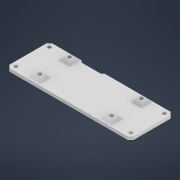
# Autodesk Inventor part: VFD_Mount
Saved by Autodesk Inventor 2021.1 (Build 251245010, 245A)
## iProperties
Created: 2020-11-26
Part Number: VFD_Mount
Material: Generic
Document SubType Name: Modeling
Designer: Alex
Density: 1 g/cm^3
Appearance: Default
Author: Alex
Autodesk Inventor part; units mm, degrees
ref_plane "YZ Plane" through (0, 0, 0) normal (1, 0, 0) x (0, 1, 0)
ref_plane "XZ Plane" through (0, 0, 0) normal (0, 1, 0) x (-1, 0, 0)
ref_plane "XY Plane" through (0, 0, 0) normal (0, 0, 1) x (1, 0, 0)
sketch "Sketch1" plane through (0, 0, 0) normal (0, 1, 0) x (-1, 0, 0)
  line L0 (64.8, -22.3) -> (-64.8, -22.3)
  line L1 (-64.8, -22.3) -> (-64.8, 22.3)
  line L2 (-64.8, 22.3) -> (64.8, 22.3)
  line L3 (64.8, 22.3) -> (64.8, -22.3)
  point P0 (0, 0)
  point P1 (64.8, 0)
  point P2 (0, -22.3)
  dimension "d0" = 129.6
  dimension "d1" = 44.6
  constraints: 8 end point, 2 midpoint, 2 parallel, 1 horizontal, 1 horizontal alignment, 1 perpendicular, 1 vertical alignment
  measures "d0" distance of L0.start L0.end
  measures "d1" distance of L2.end L0.start
extrude "Extrusion1" add sketch "Sketch1" along normal blind 3
sketch "Sketch2" plane through (0, 3, 0) normal (0, 1, 0) x (1, 0, 0)
  line L0 (-64.8, -22.3) -> (64.8, -22.3) construction
  line L1 (64.8, -22.3) -> (64.8, 22.3) construction
  line L2 (64.8, 22.3) -> (-64.8, 22.3) construction
  line L3 (-64.8, 22.3) -> (-64.8, -22.3) construction
  line L4 (-40, 18.55) -> (40, 18.55) construction
  line L5 (40, 18.55) -> (40, -17.45) construction
  line L6 (40, -17.45) -> (-40, -17.45) construction
  line L7 (-40, -17.45) -> (-40, 18.55) construction
  circle A0 centre (-37.5, 16.05) radius 1.25 construction
  circle A1 centre (37.5, 16.05) radius 1.25 construction
  circle A2 centre (37.5, -14.95) radius 1.25 construction
  circle A3 centre (-37.5, -14.95) radius 1.25 construction
  line L8 (-37.5, 12.5) -> (37.5, 12.5) construction
  line L9 (37.5, 12.5) -> (37.5, -12.5) construction
  line L10 (37.5, -12.5) -> (-37.5, -12.5) construction
  line L11 (-37.5, -12.5) -> (-37.5, 12.5) construction
  line L12 (-40, 18.55) -> (-35, 18.55)
  line L13 (-35, 18.55) -> (-35, 13.55)
  line L14 (-35, 13.55) -> (-40, 13.55)
  line L15 (-40, 13.55) -> (-40, 18.55)
  line L16 (-40, 18.55) -> (-35, 13.55) construction
  line L17 (-35, 18.55) -> (-40, 13.55) construction
  line L18 (35, 18.55) -> (40, 18.55)
  line L19 (40, 18.55) -> (40, 13.55)
  line L20 (40, 13.55) -> (35, 13.55)
  line L21 (35, 13.55) -> (35, 18.55)
  line L22 (35, 18.55) -> (40, 13.55) construction
  line L23 (40, 18.55) -> (35, 13.55) construction
  line L24 (35, -12.45) -> (40, -12.45)
  line L25 (40, -12.45) -> (40, -17.45)
  line L26 (40, -17.45) -> (35, -17.45)
  line L27 (35, -17.45) -> (35, -12.45)
  line L28 (35, -12.45) -> (40, -17.45) construction
  line L29 (40, -12.45) -> (35, -17.45) construction
  line L30 (-40, -12.45) -> (-35, -12.45)
  line L31 (-35, -12.45) -> (-35, -17.45)
  line L32 (-35, -17.45) -> (-40, -17.45)
  line L33 (-40, -17.45) -> (-40, -12.45)
  line L34 (-40, -12.45) -> (-35, -17.45) construction
  line L35 (-35, -12.45) -> (-40, -17.45) construction
  point P0 (0, 0)
  point P1 (0, 12.5)
  point P2 (0, 22.3)
  dimension "d4" = 80
  dimension "d5" = 36
  dimension "d6" = 2.5
  dimension "d7" = 2.5
  dimension "d8" = 2.5
  dimension "d9" = 2.5
  dimension "d10" = 2.5
  dimension "d12" = 75
  dimension "d13" = 25
  dimension "d14" = 2.5
  dimension "d15" = 4.95
  dimension "d16" = 9.8
  dimension "d17" = 5
  constraints: 64 end point, 12 parallel, 10 midpoint, 7 equal length, 6 horizontal, 6 perpendicular, 4 centre point, 3 equal radius, 3 vertical alignment, 2 horizontal alignment
  measures "d4" distance of L5.end L6.end
  measures "d5" distance of L4.end L5.end
  measures "d6" diameter of A0
  measures "d7" distance from line of L7 A0.centre
  measures "d8" distance from line of A1.centre L5
  measures "d9" distance from line of L4 A0.centre
  measures "d10" distance from line of L6 A3.centre
  measures "d12" distance of L8.start L8.end
  measures "d13" distance of L10.end L8.start
  measures "d14" distance between parallel lines of L7 L11
  measures "d15" distance between parallel lines of L10 L6
  measures "d16" distance between parallel lines of L10 L0
  measures "d17" distance of L12.end L13.end
extrude "Extrusion2" add sketch "Sketch2" along normal blind 3
sketch "Sketch3" plane through (0, 6, 0) normal (0, 1, 0) x (1, 0, 0)
  line L0 (-35, 18.55) -> (-40, 13.55) construction
  point P0 (0, 0)
  point P1 (-37.5, -14.95)
  point P2 (-37.5, 16.05)
  point P3 (37.5, 16.05)
  point P4 (37.5, -14.95)
hole "Hole1" at (-37.5, 6, 14.95) at (-37.5, 6, -16.05) at (37.5, 6, -16.05) at (37.5, 6, 14.95) direction (0, -1, 0) diameter 3.5 depth 4
chamfer "Chamfer1" distance 3 angle 45 16 edges at (-37.5, 3, -13.55) (-40, 3, -16.05) (-37.5, 3, -18.55) (-35, 3, -16.05) (-37.5, 3, 12.45) (-40, 3, 14.95) (-37.5, 3, 17.45) (-35, 3, 14.95) (37.5, 3, -13.55) (35, 3, -16.05) (37.5, 3, -18.55) (40, 3, -16.05) (37.5, 3, 12.45) (35, 3, 14.95) (37.5, 3, 17.45) (40, 3, 14.95)
sketch "Sketch4" plane through (0, 3, 0) normal (0, 1, 0) x (1, 0, 0)
  line L0 (43, 10.55) -> (43, 21.55) construction
  line L1 (32, 10.55) -> (43, 10.55) construction
  line L2 (32, 21.55) -> (32, 10.55) construction
  line L3 (43, 21.55) -> (32, 21.55) construction
  line L4 (-32, 10.55) -> (-32, 21.55) construction
  line L5 (-43, 10.55) -> (-32, 10.55) construction
  line L6 (-43, 21.55) -> (-43, 10.55) construction
  line L7 (-32, 21.55) -> (-43, 21.55) construction
  line L8 (-64.8, -22.3) -> (64.8, -22.3) construction
  line L9 (64.8, -22.3) -> (64.8, 22.3) construction
  line L10 (64.8, 22.3) -> (-64.8, 22.3) construction
  line L11 (-64.8, 22.3) -> (-64.8, -22.3) construction
  line L12 (-43, -9.45) -> (-43, -20.45) construction
  line L13 (-32, -9.45) -> (-43, -9.45) construction
  line L14 (-32, -20.45) -> (-32, -9.45) construction
  line L15 (-43, -20.45) -> (-32, -20.45) construction
  line L16 (32, -9.45) -> (32, -20.45) construction
  line L17 (43, -9.45) -> (32, -9.45) construction
  line L18 (43, -20.45) -> (43, -9.45) construction
  line L19 (32, -20.45) -> (43, -20.45) construction
  line L20 (64.8, 22.3) -> (-64.8, 22.3) construction
  line L21 (-31, 22.3) -> (-29, 20.3)
  line L22 (-29, 20.3) -> (-9, 20.3)
  line L23 (-9, 20.3) -> (-7, 22.3)
  line L24 (-31, 22.3) -> (-7, 22.3)
  point P0 (0, 0)
  dimension "d31" = 2
  dimension "d32" = 20
  dimension "d33" = 135
  dimension "d34" = 135
  dimension "d35" = 1
  constraints: 8 end point, 2 point on line, 1 collinear, 1 parallel
  measures "d31" distance between parallel lines of L10 L22
  measures "d32" distance of L22.end L21.end
  measures "d33" angle of L22 L21
  measures "d34" angle of L23 L22
  measures "d35" horizontal distance of L21.start L4.end
extrude "Extrusion3" cut sketch "Sketch4" against normal blind 3
chamfer "Chamfer2" distance 3 angle 45 4 edges at (-64.8, 1.5, -22.3) (-64.8, 1.5, 22.3) (64.8, 1.5, 22.3) (64.8, 1.5, -22.3)
sketch "Sketch5" plane through (0, 3, 0) normal (0, 1, 0) x (1, 0, 0)
  line L0 (43, 10.55) -> (43, 21.55) construction
  line L1 (32, 10.55) -> (43, 10.55) construction
  line L2 (32, 21.55) -> (32, 10.55) construction
  line L3 (43, 21.55) -> (32, 21.55) construction
  line L4 (-32, 10.55) -> (-32, 21.55) construction
  line L5 (-43, 10.55) -> (-32, 10.55) construction
  line L6 (-43, 21.55) -> (-43, 10.55) construction
  line L7 (-32, 21.55) -> (-43, 21.55) construction
  line L8 (-43, -9.45) -> (-43, -20.45) construction
  line L9 (-32, -9.45) -> (-43, -9.45) construction
  line L10 (-32, -20.45) -> (-32, -9.45) construction
  line L11 (-43, -20.45) -> (-32, -20.45) construction
  line L12 (32, -9.45) -> (32, -20.45) construction
  line L13 (43, -9.45) -> (32, -9.45) construction
  line L14 (43, -20.45) -> (43, -9.45) construction
  line L15 (32, -20.45) -> (43, -20.45) construction
  line L16 (61.8, 22.3) -> (64.8, 19.3) construction
  line L17 (61.8, 22.3) -> (-7, 22.3) construction
  line L18 (-7, 22.3) -> (-9, 20.3) construction
  line L19 (-9, 20.3) -> (-29, 20.3) construction
  line L20 (-29, 20.3) -> (-31, 22.3) construction
  line L21 (-31, 22.3) -> (-61.8, 22.3) construction
  line L22 (-64.8, 19.3) -> (-61.8, 22.3) construction
  line L23 (-64.8, 19.3) -> (-64.8, -19.3) construction
  line L24 (-61.8, -22.3) -> (-64.8, -19.3) construction
  line L25 (-61.8, -22.3) -> (61.8, -22.3) construction
  line L26 (64.8, -19.3) -> (61.8, -22.3) construction
  line L27 (64.8, -19.3) -> (64.8, 19.3) construction
  point P0 (0, 0)
  point P1 (-60, 17.5)
  point P2 (-60, -17.5)
  point P3 (60, -17.5)
  point P4 (60, 17.5)
  dimension "d49" = 4.8
  dimension "d50" = 4.8
  dimension "d51" = 4.8
  dimension "d52" = 4.8
  constraints: 2 horizontal alignment, 2 vertical alignment
  measures "d49" distance from line of point (-60, 17.5) L23
  measures "d50" distance from line of L21 point (-60, 17.5)
  measures "d51" distance from line of point (-60, -17.5) L25
  measures "d52" distance from line of point (60, 17.5) L27
hole "Hole2" at (-60, 3, -17.5) at (-60, 3, 17.5) at (60, 3, 17.5) at (60, 3, -17.5) direction (0, -1, 0) diameter 3.4 depth 4 clearance for "Hex Head Cap Screw ISO 24017" size "M3" standard "ISO"
equation "\"d8\" = d7"
equation "\"d9\" = d7"
equation "\"d10\" = d7"
equation "\"d34\" = d33"
equation "\"d49\" = d50"
equation "\"d51\" = d50"
equation "\"d52\" = d50"
body "Solid1"
